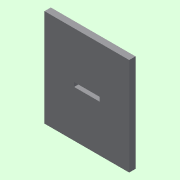
# Autodesk Inventor part: Distance_test_adaptor_slit_1mm
Saved by Autodesk Inventor 2015 (Build 190159000, 159)
## iProperties
Created: 2015-05-18
Part Number: Distance_test_adaptor_slit_1mm
Material: Generic
Document SubType Name: Modeling
Designer: Openlab
Density: 1 g/cm^3
Appearance: Default
Author: Openlab
Autodesk Inventor part; units mm, degrees
ref_plane "YZ Plane" through (0, 0, 0) normal (1, 0, 0) x (0, 1, 0)
ref_plane "XZ Plane" through (0, 0, 0) normal (0, 1, 0) x (-1, 0, 0)
ref_plane "XY Plane" through (0, 0, 0) normal (0, 0, 1) x (1, 0, 0)
sketch "Sketch1" plane through (0, 0, 0) normal (0, 1, 0) x (-1, 0, 0)
  line L0 (0, 0) -> (0, -23)
  line L1 (0, -23) -> (20, -23)
  line L2 (20, -23) -> (20, 0)
  line L3 (16.0214, -11.5) -> (3.8301, -11.5) construction
  line L4 (20, 0) -> (0, 0)
  line L5 (13, -11) -> (7, -11)
  line L6 (7, -11) -> (7, -12)
  line L7 (7, -12) -> (13, -12)
  line L8 (13, -12) -> (13, -11)
  line L9 (10, -8) -> (10, -15) construction
  dimension "d0" = 23
  dimension "d10" = 20
  dimension "d13" = 10
  dimension "d14" = 1
  dimension "d15" = 6
  constraints: 20 end point, 3 horizontal, 2 parallel, 2 perpendicular, 2 vertical, 3 other
  measures "d0" distance of L0.end L0.start
  measures "d10" distance of L2.end L0.start
  measures "d13" distance between parallel lines of L2 L9
  measures "d14" distance of L5.end L6.end
  measures "d15" distance of L5.start L5.end
extrude "Extrusion4" add sketch "Sketch1" along normal blind 1.5
body "Solid3"
